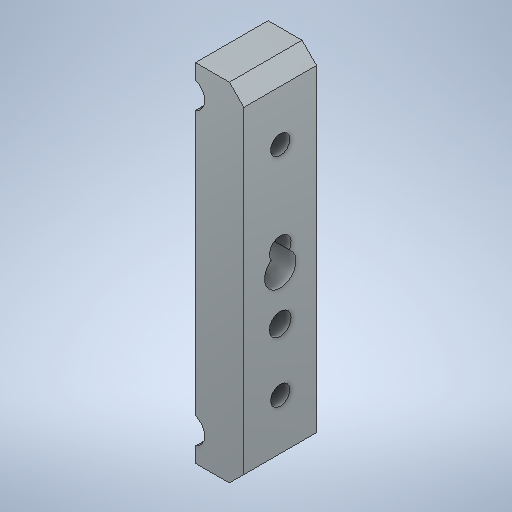
# Autodesk Inventor part: 6xMounting_base
Saved by Autodesk Inventor 2025.1 (Build 291241000, 241)
## iProperties
Created: 2024-11-24
Part Number: 6xMounting_base
Material: Ogólny
Document SubType Name: Modeling
Designer: zychlix
Density: 1 g/cm^3
Appearance: Domyślna
Author: zychlix
Autodesk Inventor part; units mm, degrees
ref_plane "YZ Plane" through (0, 0, 0) normal (1, 0, 0) x (0, 1, 0)
ref_plane "XZ Plane" through (0, 0, 0) normal (0, 1, 0) x (-1, 0, 0)
sketch "Szkic1" plane through (0, 0, 0) normal (0, 0, 1) x (1, 0, 0)
  arc A0 (3, 14.9136) -> (3, 9.2591) centre (3.6454, 12.0864) ccw projected
  circle A1 centre (3.6454, 12.0864) radius 2.9
  line L0 (4.6454, 14.8085) -> (4.6454, 17.9136)
  line L1 (3, 17.9136) -> (0, 17.9136) projected
  line L2 (4.6454, 17.9136) -> (11.6454, 17.9136)
  line L3 (14.6454, 14.9136) -> (14.6454, -17.9136)
  line L4 (-2.916, -17.9136) -> (18.8782, -17.9136) construction
  line L5 (4.6454, 9.3642) -> (4.6454, -17.9136)
  line L6 (4.6454, -17.9136) -> (14.6454, -17.9136)
  line L7 (11.6454, 17.9136) -> (14.6454, 14.9136)
  point P0 (0, 0)
  dimension "d0" = 45
  dimension "d1" = 3
  dimension "d8" = 30
  dimension "d9" = 1
  dimension "d10" = 5.8
  dimension "d11" = 11
  constraints: 14 end point, 3 perpendicular, 3 point on line, 2 horizontal, 2 point on circle, 1 centre point, 1 coincident, 1 collinear, 1 vertical
  measures "d0" angle of L2 L7
  measures "d1" distance from line of L2.end L3
  measures "d8" distance from line of A0.centre L4
  measures "d9" distance from line of L0 A0.centre
  measures "d10" diameter of A1
  measures "d11" distance from line of L3 A0.centre
ref_plane "Płaszczyzna konstrukcyjna1" through (-3, -53.7409, -15) normal (0, 0, -1) x (0, 1, 0)
extrude "Wyciągnięcie proste1" add sketch "Szkic1" against normal up to surface (15 mm away) contours L0 L2 L7 L3 L6 L5 A1
mirror "Odbij1" about plane through (14.6454, -17.9136, 0) normal (0, -1, 0) of "Wyciągnięcie proste1"
sketch "Szkic2" plane through (14.6454, 14.9136, 0) normal (1, 0, 0) x (0, 0, -1)
  circle A0 centre (7.5, -10.4312) radius 2.1 construction
  circle A1 centre (7.5, -32.8273) radius 3.25 construction
  circle A2 centre (7.5, -55.2233) radius 2.1 construction
  circle A3 centre (7.5, -10.4312) radius 1.975
  circle A4 centre (7.5, -55.2233) radius 1.975
  circle A5 centre (7.5, -32.8273) radius 3.25
  circle A6 centre (7.5, -28.9673) radius 2.25
  circle A7 centre (7.5, -42.4703) radius 2.25
  line L0 (7.5, -28.9673) -> (7.5, -36.6873) construction
  line L1 (15, 0) -> (15, -65.6545) construction
  point P0 (0, -14.9136)
  dimension "d5" = 3.95
  dimension "d12" = 4.5
  dimension "d13" = 4.5
  dimension "d14" = 13.503
  dimension "d15" = 9.643
  constraints: 5 centre point, 4 coincident, 2 end point, 2 equal radius, 1 midpoint, 1 parallel, 1 point on line, 1 vertical
  measures "d5" diameter of A3
  measures "d12" diameter of A6
  measures "d13" diameter of A7
  measures "d14" distance of A7.centre L0.start
  measures "d15" distance of A7.centre A1.centre
extrude "Wyciągnięcie proste2" cut sketch "Szkic2" against normal through all
